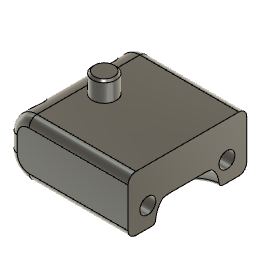
single chanel spring puller (Autodesk Fusion 360 archive; units mm, degrees)
design "end bit"
Autodesk Fusion 360 part; units mm, degrees
sketch "Sketch1" plane through (0, 0, 0) normal (0, 0, 1) x (1, 0, 0)
  line L0 (0, 0) -> (30, 0)
  line L1 (30, 0) -> (30, 30)
  line L2 (30, 30) -> (0, 30)
  line L3 (0, 30) -> (0, 0)
  dimension "d1" = 30
  dimension "d2" = 30
  constraint horizontal L0
  constraint vertical L1
  constraint horizontal L2
  constraint vertical L3
  constraint coincident L0.start L3.end
  measures "d1" distance of L0.start L0.end
  measures "d2" distance of L0.start L2.end
extrude "Extrude1" add sketch "Sketch1" along normal blind 14
sketch "Sketch2" plane through (0, 0, 0) normal (-1, 0, 0) x (0, -1, 0)
  line L0 (-30, 0) -> (0, 0)
  line L1 (0, 0) -> (0, 14)
  line L2 (0, 14) -> (-30, 14)
  line L3 (-30, 14) -> (-30, 0)
  circle A0 centre (-25, 8.975) radius 2.025
  circle A1 centre (-5, 8.975) radius 2.025
  line L4 (-25, 8.975) -> (-25, 11) construction
  line L5 (-5, 8.975) -> (-5, 11) construction
  dimension "d6" = 4.05
  dimension "d7" = 4.05
  dimension "d29" = 3
  dimension "d30" = 3
  constraint coincident A0.centre L4.start
  constraint coincident A0 L4.end
  constraint parallel L1 L4
  constraint coincident A1.centre L5.start
  constraint coincident A1 L5.end
  constraint parallel L1 L5
  measures "d6" diameter of A0
  measures "d7" diameter of A1
  measures "d29" distance of L2 L4.end
  measures "d30" distance of L2 L5.end
extrude "Extrude2" cut sketch "Sketch2" against normal blind 17 contours A0 | A1
fillet "Fillet1" radius 5 2 edges at (30, 15, 14) (30, 15, 0)
fillet "Fillet2" radius 2 10 edges at (12.5, 30, 0) (28.5355, 30, 1.4645) (30, 30, 7) (28.5355, 30, 12.5355) (12.5, 30, 14) (12.5, 0, 14) (28.5355, 0, 12.5355) (30, 0, 7) (28.5355, 0, 1.4645) (12.5, 0, 0)
sketch "Sketch4" plane through (0, 0, 14) normal (0, 0, 1) x (-1, 0, 0)
  line L0 (0, -2) -> (-25, -2)
  line L1 (-25, -28) -> (0, -28)
  line L2 (0, -28) -> (0, -2)
  circle A0 centre (-30, -24) radius 2
  circle A1 centre (-30, -6) radius 2
  line L3 (-25, -2) -> (-25, -28)
  dimension "d14" = 4
  dimension "d15" = 4
  measures "d14" diameter of A0
  measures "d15" diameter of A1
extrude "Extrude3" cut sketch "Sketch4" against normal blind 15 contours A0 | A1
fillet "Fillet3" radius 1 8 edges at (30, 26, 7) (28, 24, 1) (30, 22, 7) (28, 24, 13) (30, 4, 7) (28, 6, 13) (30, 8, 7) (28, 6, 1)
sketch "Sketch5" plane through (0, 0, 14) normal (0, 0, 1) x (-1, 0, 0)
  line L0 (0, -2) -> (-25, -2)
  line L1 (-25, -28) -> (0, -28)
  line L2 (0, -28) -> (0, -2)
  arc A0 (0, -7) -> (0, -23) centre (1.0714, -15) ccw
  line L3 (-25, -2) -> (-25, -28)
  constraint coincident L2 A0.start
  constraint coincident L2 A0.end
extrude "Extrude4" cut sketch "Sketch5" against normal blind 5 contours L2 A0
fillet "Fillet5" radius 1 1 edges at (7, 15, 14)
chamfer "Chamfer1" distance 2 angle 45 1 edges at (7, 15, 9)
fillet "Fillet6" radius 6 2 edges at (7, 15, 11) (5, 15, 9)
sketch "Sketch6" plane through (0, 0, 0) normal (0, 0, -1) x (1, 0, 0)
  line L0 (25, -2) -> (0, -2)
  line L1 (0, -2) -> (0, -28)
  line L2 (0, -28) -> (25, -28)
  line L3 (25, -28) -> (25, -2)
  circle A0 centre (17, -20) radius 2.5
  line L4 (0, -30) -> (25, -30)
  circle A1 centre (17, -10) radius 2.5
  line L5 (25, 0) -> (0, 0)
  dimension "d31" = 5
  dimension "d32" = 10
  dimension "d33" = 17
  dimension "d34" = 5
  dimension "d35" = 10
  dimension "d36" = 17
  measures "d31" diameter of A0
  measures "d32" distance of A0.centre L4
  measures "d33" distance of L1 A0.centre
  measures "d34" diameter of A1
  measures "d35" distance of A1.centre L5
  measures "d36" distance of L1 A1.centre
sketch "Sketch7" plane through (0, 30, 0) normal (0, 1, 0) x (-1, 0, 0)
  line L0 (-25, 2) -> (0, 2)
  line L1 (0, 2) -> (0, 12)
  line L2 (0, 12) -> (-25, 12)
  arc A0 (-25, 12) -> (-28, 9) centre (-25, 9) ccw
  line L3 (-28, 9) -> (-28, 5)
  arc A1 (-28, 5) -> (-25, 2) centre (-25, 5) ccw
  line L4 (-19.5, 0) -> (-19.5, -1.5)
  line L5 (-18, -1.5) -> (-18, -3)
  line L6 (-19.5, -3) -> (-19.5, -1.5)
  line L7 (-19.5, -3) -> (-19.5, -4.5)
  line L8 (-19.5, -4.5) -> (-18, -3)
  line L9 (-18, -1.5) -> (-19.5, 0)
  dimension "d39" = 1.5
  constraint vertical L4
  constraint vertical L5
  constraint vertical L6
  measures "d39" distance of L4.start L4.end
move_body "Move1" bodies 1 to x (-1, 0, 0) y (0, 1, 0) z (0, 0, -1) at (50, 0, 18)
move_body "Move2" bodies 1 to x (1, 0, 0) y (0, 1, 0) z (0, 0, 1) at (0, 0, -4)
sketch "Sketch8" plane through (0, 0, 14) normal (0, 0, 1) x (-1, 0, 0)
  line L0 (-50, -28) -> (-25, -28)
  line L1 (-25, -28) -> (-25, -2)
  line L2 (-25, -2) -> (-50, -2)
  line L3 (-50, -2) -> (-50, -28)
  circle A0 centre (-29, -15) radius 3
  dimension "d44" = 6
  measures "d44" diameter of A0
extrude "Extrude7" add sketch "Sketch8" along normal blind 5 contours A0
sketch "Sketch9" plane through (0, 30, 0) normal (0, 1, 0) x (-1, 0, 0)
  line L0 (-25, 12) -> (-50, 12)
  line L1 (-50, 12) -> (-50, 2)
  line L2 (-50, 2) -> (-25, 2)
  arc A0 (-25, 2) -> (-22, 5) centre (-25, 5) ccw
  line L3 (-22, 5) -> (-22, 9)
  arc A1 (-22, 9) -> (-25, 12) centre (-25, 9) ccw
  line L4 (-26, 14) -> (-27, 15)
  line L5 (-27, 15) -> (-27, 16)
  line L6 (-27, 16) -> (-26, 17)
  line L7 (-26, 17) -> (-26, 14)
  constraint vertical L5
  constraint parallel L5 L7
extrude "Extrude8" cut sketch "Sketch9" against normal blind 35 contours L4 L5 L6 L7
chamfer "Chamfer2" distance 0.5 angle 45 1 edges at (31.797, 16.0848, 19)

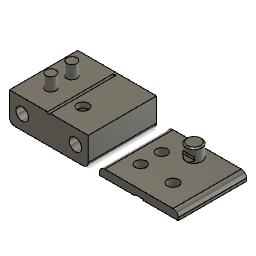
design "new pipette holder"
Autodesk Fusion 360 part; units mm, degrees
sketch "Sketch1" plane through (0, 0, 0) normal (0, 1, 0) x (1, 0, 0)
  line L0 (0, 0) -> (30, 0)
  line L1 (30, 0) -> (30, 25)
  line L2 (30, 25) -> (0, 25)
  line L3 (0, 25) -> (0, 0)
  dimension "d1" = 30
  dimension "d2" = 25
  constraint horizontal L0
  constraint vertical L1
  constraint horizontal L2
  constraint vertical L3
  constraint coincident L0.start L3.end
  measures "d1" distance of L0.start L0.end
  measures "d2" distance of L0.start L2.end
extrude "Extrude1" add sketch "Sketch1" along normal blind 11 makes body 1
sketch "Sketch2" plane through (0, 0, 0) normal (0, 0, 1) x (1, 0, 0)
  line L0 (0, 0) -> (30, 0)
  line L1 (30, 0) -> (30, 11)
  line L2 (30, 11) -> (0, 11)
  line L3 (0, 11) -> (0, 0)
  line L4 (0, 11) -> (30, 0) construction
  circle A0 centre (4.876, 5.5) radius 2.375
  line L5 (15, 5.5) -> (15, 11) construction
  circle A1 centre (25.124, 5.5) radius 2.375
  line L6 (4.876, 5.5) -> (2.501, 5.5) construction
  dimension "d5" = 4.75
  dimension "d59" = 2.501
  constraint coincident L2.end L3.start
  constraint coincident L0.end L1.start
  constraint midpoint L4 L5.start
  constraint midpoint L2 L5.end
  constraint symmetric A0 L5 A1
  constraint coincident A0.centre L6.start
  constraint coincident A0 L6.end
  constraint parallel L2 L6
  measures "d5" diameter of A0
  measures "d59" distance of L3 L6.end
extrude "Extrude2" cut sketch "Sketch2" against normal blind 36 contours A0 bodies 1
sketch "Sketch3" plane through (0, 0, 0) normal (0, 0, 1) x (1, 0, 0)
  circle A0 centre (4.876, 5.5) radius 2.375
  line L0 (0, 0) -> (30, 0)
  line L1 (30, 0) -> (30, 11)
  line L2 (30, 11) -> (0, 11)
  line L3 (0, 11) -> (0, 0)
  line L4 (14.5, 11) -> (15.5, 11)
  line L5 (15.5, 11) -> (15.5, 10.5)
  line L6 (14.5, 10.4989) -> (14.5, 11)
  arc A1 (14.5, 10.5011) -> (15.5, 10.5) centre (15, 10.5) ccw
  constraint horizontal L4
  constraint vertical L5
  constraint vertical L6
  constraint coincident L2 L4.start
  constraint tangent L5 A1
  constraint coincident L6.start A1
  constraint coincident L6 A1.start
extrude "Extrude3" cut sketch "Sketch3" against normal blind 25 contours L2 L4 L5 L6 A1 bodies 1
sketch "Sketch4" plane through (0, 11, 0) normal (0, 1, 0) x (-1, 0, 0)
  line L0 (-15.5, 0) -> (-30, 0)
  line L1 (-30, 0) -> (-30, -25)
  line L2 (-30, -25) -> (-15.5, -25)
  line L3 (-15.5, -25) -> (-30, 0) construction
  line L4 (-30, -25) -> (-15.5, 0) construction
  circle A0 centre (-19.5, -8.5) radius 2.15
  line L5 (-15.5, -25) -> (-15.5, 0)
  dimension "d12" = 4.3
  dimension "d107" = 10.5
  constraint coincident L2.end L3.start
  constraint coincident L0.end L1.start
  constraint coincident L1.end L2.start
  constraint coincident L0.start L4.end
  measures "d12" diameter of A0
  measures "d107" distance of L1 A0.centre
extrude "Extrude4" cut sketch "Sketch4" against normal blind 30 contours A0 bodies 1
sketch "Sketch5" plane through (0, 11, 0) normal (0, 1, 0) x (-1, 0, 0)
  line L0 (-14.5, -25) -> (0, -25)
  line L1 (0, -25) -> (0, 0)
  line L2 (0, 0) -> (-14.5, 0)
  line L3 (-10, -12.5) -> (1.5, -12.5) construction
  line L4 (0, -25) -> (-14.5, 0) construction
  line L5 (-7.25, -12.5) -> (-7.25, -26) construction
  circle A0 centre (-7.25, -8.5) radius 1.9
  circle A1 centre (-7.25, -16.5) radius 1.9
  line L6 (-14.5, 0) -> (-14.5, -25)
  dimension "d80" = 3.8
  dimension "d83" = 8.5
  dimension "d84" = 7.25
  constraint perpendicular L1 L3
  constraint coincident L0.end L1.start
  constraint coincident L2.end L4.end
  constraint midpoint L4 L5.start
  constraint perpendicular L0 L5
  constraint symmetric L3 A0 A1
  measures "d80" diameter of A0
  measures "d83" distance of L0 A1.centre
  measures "d84" distance of L1 A1.centre
extrude "Extrude5" add sketch "Sketch5" along normal blind 5 contours A0 bodies 1
sketch "Sketch7" plane through (0, 11, 0) normal (0, 1, 0) x (-1, 0, 0)
  circle A0 centre (-19.5, -8.5) radius 2.15
  line L0 (-15.5, 0) -> (-30, 0)
  line L1 (-30, 0) -> (-30, -25)
  line L2 (-30, -25) -> (-15.5, -25)
  line L3 (-9, -19.5) -> (-33.5, -19.5) construction
  circle A1 centre (-20, -20.5) radius 2.5
  line L4 (-15.5, -25) -> (-15.5, 0)
  constraint perpendicular L1 L3
sketch "Sketch8" plane through (0, 0, 0) normal (0, -1, 0) x (1, 0, 0)
  circle A0 centre (19.5, -8.5) radius 2.15
  line L0 (0, 0) -> (0, -25)
  line L1 (0, -25) -> (30, -25)
  line L2 (30, -25) -> (30, 0)
  line L3 (30, 0) -> (0, 0)
  line L4 (23.6498, -8.4608) -> (21.541, -4.8866)
  line L5 (21.541, -4.8866) -> (17.3912, -4.9257)
  line L6 (17.3912, -4.9257) -> (15.3502, -8.5392)
  line L7 (15.3502, -8.5392) -> (17.459, -12.1134)
  line L8 (17.459, -12.1134) -> (21.6088, -12.0743)
  line L9 (21.6088, -12.0743) -> (23.6498, -8.4608)
  point P0 (19.5, -8.5)
  dimension "d27" = 4.15
  constraint coincident P0 A0.centre
  measures "d27" distance of L4.start P0
extrude "Extrude8" cut sketch "Sketch8" against normal blind 9 contours L4 L5 L6 L7 L8 L9 bodies 1
ref_plane "WorkPlane1" through (7.25, 29, -12.5) normal (0, 1, 0) x (0, 0, 1) in component "top bit"
sketch "Sketch1 (2)" plane through (0, 29, 0) normal (0, 1, 0) x (1, 0, 0) in component "top bit"
  line L0 (0, 25) -> (30, 25)
  line L1 (30, 25) -> (30, 0)
  line L2 (30, 0) -> (0, 0)
  line L3 (0, 0) -> (0, 25)
  constraint horizontal L0
  constraint vertical L1
  constraint horizontal L2
  constraint vertical L3
extrude "Extrude1'" add sketch "Sketch1 (2)" along normal blind 3 separate body makes body 2 in component "top bit"
sketch "Sketch3 (2)" plane through (0, 0, 0) normal (0, 0, 1) x (1, 0, 0) in component "top bit"
  line L0 (0, 29) -> (30, 29)
  line L1 (30, 29) -> (30, 32)
  line L2 (30, 32) -> (0, 32)
  line L3 (0, 32) -> (0, 29)
  line L4 (15, 11) -> (15, 37.4734) construction
  circle A0 centre (15, 29) radius 0.5
  dimension "d43" = 1
  constraint perpendicular L2 L4
  constraint midpoint L0 A0.centre
  measures "d43" diameter of A0
extrude "Extrude5'" cut sketch "Sketch3 (2)" against normal blind 100 contours L0 A0 picked at (15.1222, 29.2116) bodies 2 in component "top bit"
move_body "Move1" bodies 2 to x (1, 0, 0) y (0, 1, 0) z (0, 0, 1) at (0, -18, 0) in component "top bit"
move_body "Move2" bodies 2 to x (-1, 0, 0) y (0, -1, 0) z (0, 0, 1) at (64.9701, 14, 0) in component "top bit"
fillet "Fillet3" radius 2 2 edges at (30, 0, -12.5) (0, 0, -12.5) on bodies 1
fillet "Fillet2" radius 2 2 edges at (34.9701, 0, -12.5) (64.9701, 0, -12.5) on bodies 2 in component "top bit"
extrude "Extrude9" add 1 faces at (24.4835, 7.0944, -25) along direction (0, 0, -1) blind 1 on bodies 1 bodies 1
sketch "Sketch9" plane through (0, 0, -26) normal (0, 0, -1) x (-1, 0, 0)
  arc A0 (-2, 0) -> (0, 2) centre (-2, 2) ccw
  line L0 (0, 2) -> (0, 11)
  line L1 (0, 11) -> (-14.5, 11)
  line L2 (-30, 11) -> (-30, 2)
  arc A1 (-30, 2) -> (-28, 0) centre (-28, 2) ccw
  line L3 (-28, 0) -> (-2, 0)
  circle A2 centre (-4.876, 5.5) radius 2.375
  arc A3 (-15.5, 11) -> (-14.5, 11) centre (-15, 11) ccw
  line L4 (-15.5, 11) -> (-14.5, 11)
  line L5 (-14.5, 11) -> (-14.5, 10.5011)
  line L6 (-15.5, 10.5) -> (-15.5, 11)
  line L7 (-15.5, 11) -> (-30, 11)
  arc A4 (-15.5, 10.5) -> (-14.5, 10.5011) centre (-15, 10.5) ccw
  constraint coincident A3.start L4.start
  constraint coincident L1.end A3.end
extrude "Extrude10" add sketch "Sketch9" against normal blind 1 contours A3 L4 bodies 1
extrude "Extrude6" add 1 faces at (40.4701, 2, -25) along direction (0, 0, -1) blind 1 on bodies 2 bodies 2 in component "top bit"
sketch "Sketch10" plane through (0, 0, -26) normal (0, 0, -1) x (-1, 0, 0)
  arc A0 (-64.9701, 2) -> (-62.9701, 0) centre (-62.9701, 2) ccw
  line L0 (-62.9701, 0) -> (-36.9701, 0)
  arc A1 (-36.9701, 0) -> (-34.9701, 2) centre (-36.9701, 2) ccw
  line L1 (-34.9701, 2) -> (-34.9701, 3)
  line L2 (-34.9701, 3) -> (-49.4701, 3)
  arc A2 (-50.4701, 3) -> (-49.4701, 3) centre (-49.9701, 3) ccw
  line L3 (-50.4701, 3) -> (-64.9701, 3)
  line L4 (-64.9701, 3) -> (-64.9701, 2)
  arc A3 (-50.4701, 3) -> (-49.4701, 3) centre (-49.9701, 3) ccw
  line L5 (-50.4701, 3) -> (-50.4, 3)
  line L6 (-50.4, 3) -> (-49.4701, 3)
  constraint concentric A2 A3
  constraint coincident A2.start L3.start
  constraint parallel L3 L5
  constraint coincident L2.end A2.end
  constraint parallel L2 L6
extrude "Extrude7" add sketch "Sketch10" against normal blind 1 contours A2 A3 L5 L6 bodies 2 in component "top bit"
extrude "Extrude11" cut sketch "Sketch2" against normal blind 60 contours A1 bodies 1
sketch "Sketch11" plane through (0, 11, 0) normal (0, 1, 0) x (-1, 0, 0)
  circle A0 centre (-7.25, -8.5) radius 1.9
  circle A1 centre (-19.5, -8.5) radius 2.15
  line L0 (-15.5, 0) -> (-30, 0)
  line L1 (-30, 0) -> (-30, -26)
  line L2 (-30, -26) -> (-15.5, -26)
  line L3 (0, -26) -> (0, 0)
  circle A2 centre (-10, -20.5) radius 2.5
  line L4 (-15.5, -26) -> (-15.5, -25)
  line L5 (-15.5, -25) -> (-15.5, 0)
  line L6 (-14.5, 0) -> (-14.5, -25)
  line L7 (-14.5, -25) -> (-14.5, -26)
  line L8 (-14.5, -26) -> (0, -26)
  line L9 (0, 0) -> (-14.5, 0)
  dimension "d62" = 5
  dimension "d63" = 10
  measures "d62" diameter of A2
  measures "d63" distance of L3 A2.centre
ref_plane "WorkPlane1" through (0, 6.5, -13) normal (-1, 0, 0) x (0, 0, 1)
sketch "Sketch12" plane through (0, 0, 0) normal (-1, 0, 0) x (0, 0, 1)
  line L0 (-18, 14.5) -> (-18, 16)
  line L1 (-19.5, 16) -> (-19.5, 17.5)
  line L2 (-18, 17.5) -> (-18, 16)
  line L3 (-18, 17.5) -> (-18, 19)
  line L4 (-18, 19) -> (-19.5, 17.5)
  line L5 (-19.5, 16) -> (-18, 14.5)
  constraint vertical L0
  constraint vertical L1
  constraint vertical L2
  constraint perpendicular L4 L5
extrude "Extrude13" cut sketch "Sketch12" against normal blind 25 bodies 1
sketch "Sketch13" plane through (0, 11, 0) normal (0, 1, 0) x (-1, 0, 0)
  circle A0 centre (-7.25, -8.5) radius 1.9
  circle A1 centre (-19.5, -8.5) radius 2.15
  line L0 (-15.5, 0) -> (-30, 0)
  line L1 (-30, 0) -> (-30, -26)
  line L2 (-30, -26) -> (-15.5, -26)
  line L3 (0, -26) -> (0, 0)
  line L4 (-15.5, -26) -> (-15.5, -25)
  line L5 (-15.5, -25) -> (-15.5, 0)
  line L6 (-14.5, 0) -> (-14.5, -25)
  line L7 (-14.5, -25) -> (-14.5, -26)
  line L8 (-14.5, -26) -> (0, -26)
  line L9 (0, 0) -> (-14.5, 0)
sketch "Sketch5 (2)" plane through (0, 3, 0) normal (0, 1, 0) x (-1, 0, 0) in component "top bit"
  line L0 (-49.4701, 0) -> (-49.4701, -25)
  line L1 (-49.4701, -25) -> (-50.4701, -25)
  line L2 (-50.4701, -25) -> (-50.4701, 0)
  line L3 (-50.4701, 0) -> (-64.9701, 0)
  line L4 (-64.9701, 0) -> (-64.9701, -26)
  line L5 (-64.9701, -26) -> (-34.9701, -26)
  line L6 (-34.9701, -26) -> (-34.9701, 0)
  line L7 (-34.9701, 0) -> (-49.4701, 0)
  circle A0 centre (-57.7201, -8.5) radius 1.95
  dimension "d75" = 3.9
  dimension "d76" = 8.5
  dimension "d77" = 7.25
  measures "d75" diameter of A0
  measures "d76" distance of L3 A0.centre
  measures "d77" distance of L2 A0.centre
sketch "Sketch14" plane through (0, 16, 0) normal (0, 1, 0) x (-1, 0, 0)
  circle A0 centre (-7.25, -8.5) radius 1.9
extrude "Extrude9'" cut sketch "Sketch5 (2)" against normal blind 4 contours A0 bodies 2 in component "top bit"
move_body "Move3" bodies 2 to x (-1, 0, 0) y (0, 1, 0) z (0, 0, -1) at (106.0914, 0, -26.1505) in component "top bit"
move_body "Move4" bodies 2 to x (1, 0, 0) y (0, 1, 0) z (0, 0, 1) at (21.1319, -7.9001, 0.1505) in component "top bit"
move_body "Move5" bodies 2 to x (1, 0, 0) y (0, 1, 0) z (0, 0, 1) at (-34, 0, 0) in component "top bit"
move_body "Move6" bodies 2 to x (1, 0, 0) y (0, 1, 0) z (0, 0, 1) at (0, 8, 0) in component "top bit"
move_body "Move7" bodies 2 to x (-1, 0, 0) y (0, 1, 0) z (0, 0, -1) at (104.0065, 0, -26) in component "top bit"
extrude "Extrude14" add sketch "Sketch5" along normal blind 5 contours A1 bodies 1
sketch "Sketch15" plane through (0, 3, 0) normal (0, 1, 0) x (-1, 0, 0)
  circle A0 centre (-31.5, -8.5) radius 1.95
  line L0 (-26.25, -26) -> (-26.25, 0)
  line L1 (-26.25, 0) -> (-52.25, 0)
  line L2 (-52.25, 0) -> (-52.25, -26)
  line L3 (-52.25, -26) -> (-26.25, -26)
  circle A1 centre (-39.25, -17.5) radius 2
  dimension "d85" = 4
  dimension "d86" = 8.5
  measures "d85" diameter of A1
  measures "d86" distance of L3 A1.centre
sketch "Sketch16" plane through (0, 3, 0) normal (0, 1, 0) x (-1, 0, 0)
  circle A0 centre (-31.5, -8.5) radius 1.95
  line L0 (-26.25, -26) -> (-26.25, 0)
  line L1 (-26.25, 0) -> (-52.25, 0)
  line L2 (-52.25, 0) -> (-52.25, -26)
  line L3 (-52.25, -26) -> (-26.25, -26)
  line L4 (-52.25, 0) -> (-26.25, -26) construction
  line L5 (-52.25, -26) -> (-39.25, -13) construction
  line L6 (-39.25, -13) -> (-39.25, -26) construction
  circle A1 centre (-39.25, -21) radius 3
  dimension "d89" = 6
  constraint coincident L1.end L2.start
  constraint coincident L0.start L3.end
  constraint coincident L2.end L3.start
  constraint midpoint L4 L5.end
  constraint perpendicular L3 L6
  constraint coincident L6 A1.centre
  measures "d89" diameter of A1
extrude "Extrude11'" add sketch "Sketch16" along normal blind 5 contours A1 sketch seen with x (-1, 0, 0) y (0, -1, 0) z (0, 0, 1) at (100.0032, 3.0999, 0) bodies 2 in component "top bit"
sketch "Sketch17" plane through (30, 0, 0) normal (1, 0, 0) x (0, 0, -1)
  line L0 (0, 2) -> (26, 2)
  line L1 (26, 2) -> (26, 11)
  line L2 (26, 11) -> (0, 11)
  line L3 (0, 11) -> (0, 2)
  line L4 (18.5, 3.5) -> (18, 3)
  line L5 (18, 3) -> (18, 5)
  line L6 (18.5, 3.5) -> (19, 4)
  line L7 (19, 4) -> (19, 4.5)
  line L8 (19, 4.5) -> (19, 5)
  line L9 (19, 5) -> (18.5, 5.5)
  line L10 (18.5, 5.5) -> (18, 6)
  line L11 (18, 6) -> (18, 5)
  constraint parallel L4 L6
  constraint parallel L5 L7
  constraint parallel L7 L8
  constraint perpendicular L6 L9
  constraint parallel L9 L10
  constraint parallel L5 L11
extrude "Extrude12" cut sketch "Sketch17" along normal blind 30.5 contours L4 L5 L6 L7 L8 L9 L10 L11 sketch seen with x (-1, 0, 0) y (0, -1, 0) z (0, 0, 1) at (100.0032, 3.0999, 0) bodies 2 in component "top bit"
extrude "Extrude15" add 1 faces at (14.8333, 11, -25.6667) along direction (0, -1, 0) blind 1.5 on bodies 1 bodies 1
sketch "Sketch18" plane through (0, 3, 0) normal (0, 1, 0) x (-1, 0, 0)
  circle A0 centre (-49.25, -21) radius 3
  line L0 (-62.25, 0) -> (-62.25, -26)
  line L1 (-62.25, -26) -> (-36.25, -26)
  line L2 (-36.25, -26) -> (-36.25, 0)
  line L3 (-36.25, 0) -> (-62.25, 0)
  circle A1 centre (-41.5, -8.5) radius 2.05
  line L4 (-10, -12.5) -> (1.5, -12.5) construction
  line L5 (-10, -12.5) -> (-68, -12.5) construction
  circle A2 centre (-41.5, -16.5) radius 2.05
  dimension "d96" = 4.1
  constraint coincident L4.start L5.start
  constraint perpendicular L0 L5
  constraint symmetric A1 L5 A2
  measures "d96" diameter of A1
extrude "Extrude13'" cut sketch "Sketch18" against normal blind 3 contours A1 sketch seen with x (-1, 0, 0) y (0, -1, 0) z (0, 0, 1) at (110.0032, 3.0999, 0) bodies 2 in component "top bit"
sketch "Sketch19" plane through (0, 0, 0) normal (0, 0, 1) x (1, 0, 0)
  arc A0 (36.25, 3) -> (34.25, 1) centre (36.25, 1) ccw
  line L0 (34.25, 1) -> (34.25, 0)
  line L1 (34.25, 0) -> (48.75, 0)
  arc A1 (49.75, 0) -> (48.75, 0) centre (49.25, 0) ccw
  line L2 (49.75, 0) -> (64.25, 0)
  line L3 (64.25, 0) -> (64.25, 1)
  arc A2 (64.25, 1) -> (62.25, 3) centre (62.25, 1) ccw
  line L4 (62.25, 3) -> (36.25, 3)
  line L5 (48.75, 0) -> (49.75, 0)
  line L6 (49.75, 0) -> (49.75, 0.5)
  line L7 (48.75, 0.5) -> (48.75, 0)
  arc A3 (49.75, 0.5) -> (48.75, 0.5) centre (49.25, 0.5) ccw
  constraint horizontal L5
  constraint vertical L6
  constraint vertical L7
  constraint coincident L1.end A1.end
  constraint midpoint A1 A3.centre
  constraint tangent L6 A3
extrude "Extrude14'" cut sketch "Sketch19" against normal blind 25 contours A1 L6 L7 A3 sketch seen with x (-1, 0, 0) y (0, -1, 0) z (0, 0, 1) at (110.0032, 3.0999, 0) bodies 2 in component "top bit"
chamfer "Chamfer1" distance 0.5 angle 45 1 edges at (57.9563, -4.9001, -22.0848) on bodies 2 in component "top bit"
extrude "Extrude15'" cut sketch "Sketch18" against normal blind 11 contours A2 sketch seen with x (-1, 0, 0) y (0, -1, 0) z (0, 0, 1) at (110.0032, 3.0999, 0) bodies 2 in component "top bit"
sketch "Sketch20" plane through (0, 0, 0) normal (0, -1, 0) x (1, 0, 0)
  circle A0 centre (41.5, -16.5) radius 2.05
  circle A1 centre (41.5, -8.5) radius 2.05
  line L0 (49.75, 0) -> (49.75, -25)
  line L1 (49.75, -25) -> (48.75, -25)
  line L2 (48.75, -25) -> (48.75, 0)
  line L3 (48.75, 0) -> (34.25, 0)
  line L4 (34.25, 0) -> (34.25, -26)
  line L5 (34.25, -26) -> (64.25, -26)
  line L6 (64.25, -26) -> (64.25, 0)
  line L7 (64.25, 0) -> (49.75, 0)
  circle A2 centre (19.5, -8.5) radius 2.15 construction
  line L8 (19.5, -8.5) -> (78, -8.5) construction
  circle A3 centre (53.75, -8.5) radius 2.15
  dimension "d108" = 4.3
  dimension "d109" = 10.5
  constraint coincident A2.centre L8.start
  constraint perpendicular L6 L8
  constraint coincident L8 A3.centre
  measures "d108" diameter of A3
  measures "d109" distance of L6 A3.centre
extrude "Extrude16" cut sketch "Sketch20" against normal blind 14 contours A3 sketch seen with x (-1, 0, 0) y (0, -1, 0) z (0, 0, 1) at (110.0032, 3.0999, 0) bodies 2 in component "top bit"
extrude "Extrude17" add 2 faces at (60.9034, 2.9779, -25) (60.7657, 2.2679, -25) along direction (0, 0, 1) blind 25 on bodies 2 bodies 2 in component "top bit"
sketch "Sketch21" plane through (0, 0, 0) normal (0, -1, 0) x (1, 0, 0)
  circle A0 centre (53.75, -8.5) radius 2.15
  circle A1 centre (41.5, -16.5) radius 2.05
  circle A2 centre (41.5, -8.5) radius 2.05
  line L0 (64.25, 0) -> (34.25, 0)
  line L1 (34.25, 0) -> (34.25, -26)
  line L2 (34.25, -26) -> (64.25, -26)
  line L3 (64.25, -26) -> (64.25, 0)
  line L4 (64.25, 0) -> (34.25, -26) construction
  line L5 (34.25, 0) -> (64.25, -26) construction
  line L6 (49.25, -13) -> (49.25, 0) construction
  line L7 (49.25, -13) -> (49.25, -26) construction
  line L8 (50.75, -26) -> (47.75, -26)
  line L9 (47.75, -26) -> (47.75, 0)
  line L10 (47.75, 0) -> (50.75, 0)
  line L11 (50.75, 0) -> (50.75, -26)
  line L12 (50.75, -26) -> (47.75, 0) construction
  line L13 (47.75, -26) -> (50.75, 0) construction
  point P0 (49.25, -13)
  dimension "d114" = 3
  constraint coincident L0.start L3.end
  constraint coincident L1.end L2.start
  constraint coincident L0.end L1.start
  constraint coincident L2.end L3.start
  constraint midpoint L4 P0
  constraint midpoint L0 L6.end
  constraint midpoint L2 L7.end
  constraint horizontal L8
  constraint perpendicular L8 L9
  constraint parallel L8 L10
  constraint parallel L9 L11
  constraint coincident L12 P0
  constraint coincident L13 P0
  constraint coincident L2 L8.start
  constraint coincident P0 L6.start
  measures "d114" distance of L9.end L10.end
extrude "Extrude18" cut sketch "Sketch21" against normal blind 0.75 contours L0 L2 L8 L9 L10 L11 sketch seen with x (-1, 0, 0) y (0, -1, 0) z (0, 0, 1) at (110.0032, 3.0999, 0) bodies 2 in component "top bit"
sketch "Sketch22" plane through (0, 0, 0) normal (0, 0, 1) x (1, 0, 0)
  circle A0 centre (25.124, 5.5) radius 2.375
  circle A1 centre (4.876, 5.5) radius 2.375
  arc A2 (0, 2) -> (2, 0) centre (2, 2) ccw
  line L0 (2, 0) -> (28, 0)
  arc A3 (28, 0) -> (30, 2) centre (28, 2) ccw
  line L1 (30, 2) -> (30, 11)
  line L2 (30, 11) -> (15.5, 11)
  line L3 (15.5, 11) -> (15.5, 10.5)
  arc A4 (14.5, 10.5011) -> (15.5, 10.5) centre (15, 10.5) ccw
  line L4 (14.5, 10.5011) -> (14.5, 11)
  line L5 (14.5, 11) -> (0, 11)
  line L6 (0, 11) -> (0, 2)
  line L7 (15.6, 10.6) -> (15.6, 11)
  line L8 (15.6, 11) -> (14.4, 11)
  line L9 (14.4, 11) -> (14.4, 10.6)
  arc A5 (14.4, 10.6008) -> (15.6, 10.6008) centre (15, 10.6) ccw
  constraint vertical L7
  constraint horizontal L8
  constraint vertical L9
  constraint coincident L2 L7.end
  constraint coincident L9.end A5
  constraint coincident L7 A5.end
  constraint coincident L9 A5.start
extrude "Extrude19" add 1 faces at (61.2532, 2.3499, -17.3333) along direction (0, 1, 0) blind 0.35 on bodies 2 bodies 2 in component "top bit"
extrude "Extrude17'" add 1 faces at (14.8333, 10.6663, -25) along direction (0, 0, 1) blind 25 on bodies 1 bodies 1
sketch "Sketch23" plane through (0, 0, 0) normal (0, 0, 1) x (1, 0, 0)
  circle A0 centre (25.124, 5.5) radius 2.375
  circle A1 centre (4.876, 5.5) radius 2.375
  arc A2 (0, 2) -> (2, 0) centre (2, 2) ccw
  line L0 (2, 0) -> (28, 0)
  arc A3 (28, 0) -> (30, 2) centre (28, 2) ccw
  line L1 (30, 2) -> (30, 11)
  line L2 (30, 11) -> (0, 11)
  line L3 (0, 11) -> (0, 2)
  circle A4 centre (15, 11) radius 0.5
  dimension "d123" = 1
  constraint midpoint L2 A4.centre
  measures "d123" diameter of A4
extrude "Extrude18'" cut sketch "Sketch23" against normal blind 25 contours L2 A4 picked at (14.8961, 10.7714) bodies 1
component "top bit" placed x (-1, 0, 0) y (0, -1, 0) z (0, 0, 1) at (110.0032, 3.0999, 0)
